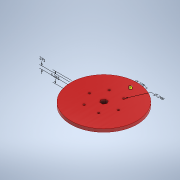
# Autodesk Inventor part: attachementToTripod
Saved by Autodesk Inventor 2022.2 (Build 262287010, 287A)
## iProperties
Created: 2021-02-15
Part Number: attachementToTripod
Material: PC/ABS Plastic
Document SubType Name: Modeling
Designer: robst
Density: 0.357273 g/cm^3
Appearance: Red
Author: robst
Autodesk Inventor part; units mm, degrees
(part 1 of 2)
ref_plane "YZ Plane" through (0, 0, 0) normal (1, 0, 0) x (0, 1, 0)
ref_plane "XZ Plane" through (0, 0, 0) normal (0, 1, 0) x (-1, 0, 0)
ref_plane "XY Plane" through (0, 0, 0) normal (0, 0, 1) x (1, 0, 0)
sketch "Sketch2" plane through (0, 0, 0) normal (0, 0, 1) x (1, 0, 0)
  line L0 (-101.6, 0) -> (-101.6, -9.525)
  line L1 (-101.6, -9.525) -> (-12.7, -9.525)
  line L2 (-10.795, -44.525) -> (0, -44.525)
  line L3 (-101.6, 0) -> (0, 0)
  line L4 (0, 0) -> (0, -44.525) construction
  line L5 (0, 0) -> (0, -44.525)
  line L6 (0, -53.43) -> (0, 8.905) projected
  line L7 (-12.7, -9.525) -> (-10.795, -44.525)
  dimension "d0" = 101.6
  dimension "d3" = 9.525
  dimension "d4" = 35
  dimension "d64" = 10.795
  constraints: 14 end point, 3 vertical, 2 horizontal, 1 perpendicular
  measures "d0" distance from line of L0 L3.end
  measures "d3" distance from line of L1 L3.end
  measures "d4" distance from line of L2.start L1
  measures "d64" horizontal distance of L2.start L3.end
revolve "Revolution1" add sketch "Sketch2" angle 360 about axis through (0, -10, 0) along (0, 1, 0)
sketch "Sketch5" plane through (0, -9.525, 0) normal (0, -1, 0) x (1, 0, 0)
  circle A0 centre (0, 0) radius 76.2 construction
  line L0 (6.8814, -79.1482) -> (6.9305, -79.1427)
  spline S0 degree 2 poles (6.9305, -79.1427) (7.0648, -79.1774) (7.5531, -79.21) (7.7433, -79.1888) knots 0 0 0 1 2 2 2
  spline S1 degree 2 poles (7.7433, -79.1888) (8.3448, -79.1218) (8.8001, -78.5243) (8.7208, -77.8124) knots 0 0 0 1 2 2 2
  line L1 (8.7208, -77.8124) -> (8.6996, -77.6221)
  line L2 (8.6996, -77.6221) -> (7.1162, -77.7986)
  line L3 (7.1162, -77.7986) -> (7.028, -77.0069)
  line L4 (7.028, -77.0069) -> (8.5807, -76.8339)
  line L5 (8.5807, -76.8339) -> (8.0356, -71.9426)
  line L6 (8.0356, -71.9426) -> (8.993, -71.8359)
  line L7 (8.993, -71.8359) -> (9.5381, -76.7272)
  line L8 (9.5381, -76.7272) -> (10.1824, -76.6554)
  line L9 (10.1824, -76.6554) -> (10.2707, -77.447)
  line L10 (10.2707, -77.447) -> (9.6263, -77.5189)
  line L11 (9.6263, -77.5189) -> (9.6475, -77.7091)
  spline S2 degree 2 poles (9.6475, -77.7091) (9.761, -78.7279) (8.8919, -79.9058) (7.9714, -80.0084) knots 0 0 0 1 2 2 2
  spline S3 degree 2 poles (7.9714, -80.0084) (7.7075, -80.0378) (7.1919, -80.0393) (6.9792, -80.0258) knots 0 0 0 1 2 2 2
  line L12 (6.9792, -80.0258) -> (6.8814, -79.1482)
  line L13 (4.5732, -72.247) -> (5.5341, -72.1798)
  line L14 (5.5341, -72.1798) -> (5.9333, -77.8839)
  line L15 (5.9333, -77.8839) -> (4.9724, -77.9511)
  line L16 (4.9724, -77.9511) -> (4.5732, -72.247)
  line L17 (4.971, -78.9045) -> (6.0613, -78.8282)
  line L18 (6.0613, -78.8282) -> (6.1312, -79.8261)
  line L19 (6.1312, -79.8261) -> (5.0408, -79.9024)
  line L20 (5.0408, -79.9024) -> (4.971, -78.9045)
  line L21 (2.1802, -72.3588) -> (3.1428, -72.3233)
  line L22 (3.1428, -72.3233) -> (3.4355, -80.2776)
  line L23 (3.4355, -80.2776) -> (2.4728, -80.313)
  line L24 (2.4728, -80.313) -> (2.1802, -72.3588)
  spline S4 degree 2 poles (-1.7121, -72.2413) (-0.3415, -72.2657) (1.1375, -73.83) (1.1122, -75.25) knots 0 0 0 1 2 2 2
  spline S5 degree 2 poles (1.1122, -75.25) (1.0873, -76.6453) (-0.4055, -78.2739) (-1.5847, -78.2528) knots 0 0 0 1 2 2 2
  spline S6 degree 2 poles (-1.5847, -78.2528) (-2.1157, -78.2433) (-2.9313, -77.92) (-3.228, -77.5874) knots 0 0 0 1 2 2 2
  spline S7 degree 2 poles (-3.228, -77.5874) (-3.5309, -77.2546) (-3.8412, -76.3042) (-3.829, -75.6188) knots 0 0 0 1 2 2 2
  line L25 (-3.829, -75.6188) -> (-3.8196, -75.094)
  line L26 (-3.8196, -75.094) -> (0.1379, -75.1647)
  spline S8 degree 2 poles (0.1379, -75.1647) (0.1557, -74.1706) (-0.8257, -73.097) (-1.7148, -73.0812) knots 0 0 0 1 2 2 2
  spline S9 degree 2 poles (-1.7148, -73.0812) (-2.0296, -73.0755) (-2.6434, -73.2066) (-2.8924, -73.3134) knots 0 0 0 1 2 2 2
  spline S10 degree 2 poles (-2.8924, -73.3134) (-3.1539, -73.4322) (-3.5158, -73.6419) (-3.6349, -73.7386) knots 0 0 0 1 2 2 2
  line L27 (-3.6349, -73.7386) -> (-3.6905, -73.7376)
  line L28 (-3.6905, -73.7376) -> (-3.6717, -72.688)
  spline S11 degree 2 poles (-3.6717, -72.688) (-3.5038, -72.6231) (-2.994, -72.4346) (-2.7955, -72.3825) knots 0 0 0 1 2 2 2
  spline S12 degree 2 poles (-2.7955, -72.3825) (-2.5162, -72.3072) (-2.0579, -72.2351) (-1.7121, -72.2413) knots 0 0 0 1 2 2 2
  spline S13 degree 2 poles (-2.8943, -75.8455) (-2.8889, -76.2347) (-2.7385, -76.8056) (-2.5876, -76.9997) knots 0 0 0 1 2 2 2
  spline S14 degree 2 poles (-2.5876, -76.9997) (-2.4247, -77.2188) (-1.904, -77.4566) (-1.515, -77.4635) knots 0 0 0 1 2 2 2
  spline S15 degree 2 poles (-1.515, -77.4635) (-1.1323, -77.4704) (-0.591, -77.2515) (-0.3648, -77.0332) knots 0 0 0 1 2 2 2
  spline S16 degree 2 poles (-0.3648, -77.0332) (-0.1446, -76.8086) (0.0874, -76.2631) (0.1248, -75.8994) knots 0 0 0 1 2 2 2
  line L29 (0.1248, -75.8994) -> (-2.8943, -75.8455)
  line L30 (-6.5023, -72.1) -> (-5.2837, -72.1995)
  line L31 (-5.2837, -72.1995) -> (-5.4023, -73.652)
  line L32 (-5.4023, -73.652) -> (-6.6209, -73.5524)
  line L33 (-6.6209, -73.5524) -> (-6.5023, -72.1)
  line L34 (-6.8491, -76.3466) -> (-5.6305, -76.4461)
  line L35 (-5.6305, -76.4461) -> (-5.7492, -77.8986)
  line L36 (-5.7492, -77.8986) -> (-6.9678, -77.7991)
  line L37 (-6.9678, -77.7991) -> (-6.8491, -76.3466)
  spline S17 degree 2 poles (-14.9177, -71.4636) (-14.7861, -71.4009) (-14.3396, -71.1724) (-14.1402, -71.1165) knots 0 0 0 1 2 2 2
  spline S18 degree 2 poles (-14.1402, -71.1165) (-13.8659, -71.031) (-13.3722, -70.9814) (-12.9477, -71.0632) knots 0 0 0 1 2 2 2
  spline S19 degree 2 poles (-12.9477, -71.0632) (-12.6021, -71.1298) (-12.0277, -71.5108) (-11.8368, -71.7928) knots 0 0 0 1 2 2 2
  spline S20 degree 2 poles (-11.8368, -71.7928) (-11.6568, -72.0664) (-11.5148, -72.7981) (-11.5872, -73.174) knots 0 0 0 1 2 2 2
  spline S21 degree 2 poles (-11.5872, -73.174) (-11.6993, -73.7562) (-12.3493, -74.4862) (-12.9284, -74.6199) knots 0 0 0 1 2 2 2
  spline S22 degree 2 poles (-12.9284, -74.6199) (-13.4434, -74.7471) (-14.7604, -74.6633) (-15.5144, -74.5621) knots 0 0 0 1 2 2 2
  line L38 (-15.5144, -74.5621) -> (-15.5495, -74.744)
  spline S23 degree 2 poles (-15.5495, -74.744) (-15.6125, -75.0714) (-15.4907, -75.5162) (-15.331, -75.6664) knots 0 0 0 1 2 2 2
  spline S24 degree 2 poles (-15.331, -75.6664) (-15.1712, -75.8167) (-14.6638, -75.9899) (-14.3849, -76.0436) knots 0 0 0 1 2 2 2
  spline S25 degree 2 poles (-14.3849, -76.0436) (-14.0574, -76.1067) (-13.1348, -76.0831) (-12.6559, -75.9804) knots 0 0 0 1 2 2 2
  line L39 (-12.6559, -75.9804) -> (-12.6013, -75.9909)
  line L40 (-12.6013, -75.9909) -> (-12.787, -76.955)
  spline S26 degree 2 poles (-12.787, -76.955) (-13.0618, -76.9776) (-14.0731, -76.9715) (-14.5521, -76.8792) knots 0 0 0 1 2 2 2
  spline S27 degree 2 poles (-14.5521, -76.8792) (-15.1342, -76.7671) (-15.8935, -76.4322) (-16.1632, -76.135) knots 0 0 0 1 2 2 2
  spline S28 degree 2 poles (-16.1632, -76.135) (-16.4281, -75.845) (-16.59, -75.0529) (-16.4884, -74.5254) knots 0 0 0 1 2 2 2
  line L41 (-16.4884, -74.5254) -> (-15.7491, -70.6871)
  line L42 (-15.7491, -70.6871) -> (-14.8032, -70.8693)
  line L43 (-14.8032, -70.8693) -> (-14.9177, -71.4636)
  line L44 (-15.0695, -72.2518) -> (-15.3696, -73.8102)
  spline S29 degree 2 poles (-15.3696, -73.8102) (-15.0242, -73.8453) (-13.9796, -73.9395) (-13.6396, -73.9044) knots 0 0 0 1 2 2 2
  spline S30 degree 2 poles (-13.6396, -73.9044) (-13.2414, -73.8616) (-12.658, -73.4772) (-12.5763, -73.0527) knots 0 0 0 1 2 2 2
  spline S31 degree 2 poles (-12.5763, -73.0527) (-12.4828, -72.5676) (-12.934, -71.9714) (-13.4554, -71.8709) knots 0 0 0 1 2 2 2
  spline S32 degree 2 poles (-13.4554, -71.8709) (-13.8981, -71.7857) (-14.6993, -72.0276) (-15.0695, -72.2518) knots 0 0 0 1 2 2 2
  spline S33 degree 2 poles (-18.707, -69.8193) (-17.9476, -70.0152) (-17.3162, -71.1028) (-17.5584, -72.0415) knots 0 0 0 1 2 2 2
  line L45 (-17.5584, -72.0415) -> (-18.3497, -75.1089)
  line L46 (-18.3497, -75.1089) -> (-17.7219, -75.2709)
  line L47 (-17.7219, -75.2709) -> (-17.9209, -76.0422)
  line L48 (-17.9209, -76.0422) -> (-18.5487, -75.8802)
  line L49 (-18.5487, -75.8802) -> (-18.959, -77.4707)
  line L50 (-18.959, -77.4707) -> (-19.8918, -77.2301)
  line L51 (-19.8918, -77.2301) -> (-19.4815, -75.6396)
  line L52 (-19.4815, -75.6396) -> (-21.1975, -75.1969)
  line L53 (-21.1975, -75.1969) -> (-20.9985, -74.4256)
  line L54 (-20.9985, -74.4256) -> (-19.2825, -74.8683)
  line L55 (-19.2825, -74.8683) -> (-18.6022, -72.2314)
  spline S34 degree 2 poles (-18.6022, -72.2314) (-18.4942, -71.8129) (-18.4054, -71.3447) (-18.4561, -71.1212) knots 0 0 0 1 2 2 2
  spline S35 degree 2 poles (-18.4561, -71.1212) (-18.4951, -70.9262) (-18.827, -70.6556) (-19.1499, -70.5723) knots 0 0 0 1 2 2 2
  spline S36 degree 2 poles (-19.1499, -70.5723) (-19.3771, -70.5137) (-19.8371, -70.5417) (-19.9436, -70.5589) knots 0 0 0 1 2 2 2
  line L56 (-19.9436, -70.5589) -> (-19.9974, -70.545)
  line L57 (-19.9974, -70.545) -> (-19.7815, -69.7079)
  spline S37 degree 2 poles (-19.7815, -69.7079) (-19.4999, -69.704) (-18.9401, -69.7591) (-18.707, -69.8193) knots 0 0 0 1 2 2 2
  spline S38 degree 2 poles (-22.0659, -68.8315) (-21.3169, -69.064) (-20.7389, -70.1809) (-21.0263, -71.1068) knots 0 0 0 1 2 2 2
  line L58 (-21.0263, -71.1068) -> (-21.9652, -74.1322)
  line L59 (-21.9652, -74.1322) -> (-21.346, -74.3244)
  line L60 (-21.346, -74.3244) -> (-21.5821, -75.0852)
  line L61 (-21.5821, -75.0852) -> (-22.2013, -74.893)
  line L62 (-22.2013, -74.893) -> (-22.6881, -76.4618)
  line L63 (-22.6881, -76.4618) -> (-23.6082, -76.1763)
  line L64 (-23.6082, -76.1763) -> (-23.1213, -74.6075)
  line L65 (-23.1213, -74.6075) -> (-24.8139, -74.0822)
  line L66 (-24.8139, -74.0822) -> (-24.5778, -73.3214)
  line L67 (-24.5778, -73.3214) -> (-22.8852, -73.8467)
  line L68 (-22.8852, -73.8467) -> (-22.0781, -71.2459)
  spline S39 degree 2 poles (-22.0781, -71.2459) (-21.95, -70.8331) (-21.8385, -70.3698) (-21.8784, -70.1441) knots 0 0 0 1 2 2 2
  spline S40 degree 2 poles (-21.8784, -70.1441) (-21.9079, -69.9474) (-22.2263, -69.6611) (-22.5448, -69.5622) knots 0 0 0 1 2 2 2
  spline S41 degree 2 poles (-22.5448, -69.5622) (-22.7689, -69.4927) (-23.2297, -69.4984) (-23.3369, -69.5104) knots 0 0 0 1 2 2 2
  line L69 (-23.3369, -69.5104) -> (-23.39, -69.4939)
  line L70 (-23.39, -69.4939) -> (-23.1338, -68.6682)
  spline S42 degree 2 poles (-23.1338, -68.6682) (-22.8523, -68.678) (-22.2959, -68.7602) (-22.0659, -68.8315) knots 0 0 0 1 2 2 2
  spline S43 degree 2 poles (-26.9866, -67.8329) (-26.8462, -67.7937) (-26.3671, -67.6455) (-26.161, -67.6247) knots 0 0 0 1 2 2 2
  spline S44 degree 2 poles (-26.161, -67.6247) (-25.8761, -67.5876) (-25.3812, -67.6238) (-24.9771, -67.7773) knots 0 0 0 1 2 2 2
  spline S45 degree 2 poles (-24.9771, -67.7773) (-24.6481, -67.9023) (-24.1479, -68.3764) (-24.0083, -68.6871) knots 0 0 0 1 2 2 2
  spline S46 degree 2 poles (-24.0083, -68.6871) (-23.8781, -68.9876) (-23.8639, -69.7328) (-23.9999, -70.0907) knots 0 0 0 1 2 2 2
  spline S47 degree 2 poles (-23.9999, -70.0907) (-24.2105, -70.6449) (-24.9763, -71.2522) (-25.5699, -71.2844) knots 0 0 0 1 2 2 2
  spline S48 degree 2 poles (-25.5699, -71.2844) (-26.0991, -71.3211) (-27.382, -71.0119) (-28.1074, -70.7826) knots 0 0 0 1 2 2 2
  line L71 (-28.1074, -70.7826) -> (-28.1732, -70.9557)
  spline S49 degree 2 poles (-28.1732, -70.9557) (-28.2916, -71.2675) (-28.2481, -71.7266) (-28.1166, -71.9021) knots 0 0 0 1 2 2 2
  spline S50 degree 2 poles (-28.1166, -71.9021) (-27.9851, -72.0775) (-27.515, -72.3354) (-27.2495, -72.4363) knots 0 0 0 1 2 2 2
  spline S51 degree 2 poles (-27.2495, -72.4363) (-26.9378, -72.5548) (-26.0248, -72.6903) (-25.5354, -72.6714) knots 0 0 0 1 2 2 2
  line L72 (-25.5354, -72.6714) -> (-25.4835, -72.6912)
  line L73 (-25.4835, -72.6912) -> (-25.8322, -73.609)
  spline S52 degree 2 poles (-25.8322, -73.609) (-26.1067, -73.5839) (-27.1019, -73.404) (-27.5579, -73.2307) knots 0 0 0 1 2 2 2
  spline S53 degree 2 poles (-27.5579, -73.2307) (-28.1121, -73.0202) (-28.8024, -72.5597) (-29.0171, -72.2205) knots 0 0 0 1 2 2 2
  spline S54 degree 2 poles (-29.0171, -72.2205) (-29.2281, -71.8893) (-29.2513, -71.0811) (-29.0605, -70.579) knots 0 0 0 1 2 2 2
  line L74 (-29.0605, -70.579) -> (-27.6721, -66.925)
  line L75 (-27.6721, -66.925) -> (-26.7716, -67.2672)
  line L76 (-26.7716, -67.2672) -> (-26.9866, -67.8329)
  line L77 (-27.2717, -68.5833) -> (-27.8354, -70.0668)
  spline S55 degree 2 poles (-27.8354, -70.0668) (-27.5012, -70.1608) (-26.4884, -70.4333) (-26.1473, -70.4572) knots 0 0 0 1 2 2 2
  spline S56 degree 2 poles (-26.1473, -70.4572) (-25.7478, -70.4835) (-25.1069, -70.2051) (-24.9534, -69.8011) knots 0 0 0 1 2 2 2
  spline S57 degree 2 poles (-24.9534, -69.8011) (-24.7779, -69.3393) (-25.1198, -68.6743) (-25.6162, -68.4857) knots 0 0 0 1 2 2 2
  spline S58 degree 2 poles (-25.6162, -68.4857) (-26.0376, -68.3256) (-26.8685, -68.426) (-27.2717, -68.5833) knots 0 0 0 1 2 2 2
  spline S59 degree 2 poles (-30.919, -65.3137) (-30.3813, -65.5632) (-29.644, -66.307) (-29.4807, -66.7912) knots 0 0 0 1 2 2 2
  spline S60 degree 2 poles (-29.4807, -66.7912) (-29.3148, -67.2699) (-29.435, -68.4531) (-29.7521, -69.1364) knots 0 0 0 1 2 2 2
  spline S61 degree 2 poles (-29.7521, -69.1364) (-30.0693, -69.8198) (-30.896, -70.6478) (-31.3601, -70.841) knots 0 0 0 1 2 2 2
  spline S62 degree 2 poles (-31.3601, -70.841) (-31.8267, -71.0397) (-32.9087, -70.9801) (-33.4352, -70.7357) knots 0 0 0 1 2 2 2
  spline S63 degree 2 poles (-33.4352, -70.7357) (-33.8609, -70.5382) (-34.5445, -69.9282) (-34.7798, -69.6284) knots 0 0 0 1 2 2 2
  line L78 (-34.7798, -69.6284) -> (-34.3249, -68.6482)
  line L79 (-34.3249, -68.6482) -> (-34.2745, -68.6716)
  spline S64 degree 2 poles (-34.2745, -68.6716) (-34.2156, -68.7942) (-34.018, -69.131) (-33.8601, -69.3336) knots 0 0 0 1 2 2 2
  spline S65 degree 2 poles (-33.8601, -69.3336) (-33.7168, -69.509) (-33.2889, -69.8778) (-33.0649, -69.9817) knots 0 0 0 1 2 2 2
  spline S66 degree 2 poles (-33.0649, -69.9817) (-32.3871, -70.2963) (-31.088, -69.6533) (-30.6539, -68.7179) knots 0 0 0 1 2 2 2
  spline S67 degree 2 poles (-30.6539, -68.7179) (-30.2302, -67.8049) (-30.5499, -66.4108) (-31.2557, -66.0832) knots 0 0 0 1 2 2 2
  spline S68 degree 2 poles (-31.2557, -66.0832) (-31.6814, -65.8857) (-32.6181, -65.8799) (-33.0424, -66.0166) knots 0 0 0 1 2 2 2
  line L80 (-33.0424, -66.0166) -> (-33.0928, -65.9932)
  line L81 (-33.0928, -65.9932) -> (-32.6379, -65.0129)
  spline S69 degree 2 poles (-32.6379, -65.0129) (-32.4805, -65.0111) (-32.0078, -65.0194) (-31.8328, -65.053) knots 0 0 0 1 2 2 2
  spline S70 degree 2 poles (-31.8328, -65.053) (-31.5775, -65.0898) (-31.1935, -65.1863) (-30.919, -65.3137) knots 0 0 0 1 2 2 2
  line L82 (-37.2051, -62.1388) -> (-36.3635, -62.6076)
  line L83 (-36.3635, -62.6076) -> (-37.95, -65.4559)
  spline S71 degree 2 poles (-37.95, -65.4559) (-38.1423, -65.8012) (-38.4081, -66.4307) (-38.4102, -66.6628) knots 0 0 0 1 2 2 2
  spline S72 degree 2 poles (-38.4102, -66.6628) (-38.4128, -66.9087) (-38.1482, -67.2964) (-37.8353, -67.4707) knots 0 0 0 1 2 2 2
  spline S73 degree 2 poles (-37.8353, -67.4707) (-37.5224, -67.645) (-36.6725, -67.6801) (-36.204, -67.5877) knots 0 0 0 1 2 2 2
  line L84 (-36.204, -67.5877) -> (-34.1247, -63.8545)
  line L85 (-34.1247, -63.8545) -> (-33.2831, -64.3233)
  line L86 (-33.2831, -64.3233) -> (-37.1563, -71.277)
  line L87 (-37.1563, -71.277) -> (-37.9979, -70.8083)
  line L88 (-37.9979, -70.8083) -> (-36.5977, -68.2944)
  spline S74 degree 2 poles (-36.5977, -68.2944) (-37.1646, -68.4239) (-38.0912, -68.3743) (-38.5012, -68.1459) knots 0 0 0 1 2 2 2
  spline S75 degree 2 poles (-38.5012, -68.1459) (-39.2348, -67.7373) (-39.5248, -66.3035) (-39.0109, -65.381) knots 0 0 0 1 2 2 2
  line L89 (-39.0109, -65.381) -> (-37.2051, -62.1388)
  spline S76 degree 2 poles (-40.3503, -59.9465) (-39.2086, -60.7053) (-38.8049, -62.8199) (-39.591, -64.0027) knots 0 0 0 1 2 2 2
  spline S77 degree 2 poles (-39.591, -64.0027) (-40.3635, -65.165) (-42.4984, -65.7332) (-43.4806, -65.0803) knots 0 0 0 1 2 2 2
  spline S78 degree 2 poles (-43.4806, -65.0803) (-43.9229, -64.7864) (-44.436, -64.0746) (-44.5068, -63.6346) knots 0 0 0 1 2 2 2
  spline S79 degree 2 poles (-44.5068, -63.6346) (-44.5828, -63.1911) (-44.3324, -62.2231) (-43.953, -61.6523) knots 0 0 0 1 2 2 2
  line L90 (-43.953, -61.6523) -> (-43.6625, -61.2151)
  line L91 (-43.6625, -61.2151) -> (-40.366, -63.4061)
  spline S80 degree 2 poles (-40.366, -63.4061) (-39.8157, -62.5781) (-40.0643, -61.145) (-40.8049, -60.6528) knots 0 0 0 1 2 2 2
  spline S81 degree 2 poles (-40.8049, -60.6528) (-41.0671, -60.4785) (-41.6549, -60.2584) (-41.9221, -60.2142) knots 0 0 0 1 2 2 2
  spline S82 degree 2 poles (-41.9221, -60.2142) (-42.2065, -60.1735) (-42.6244, -60.1553) (-42.7768, -60.1726) knots 0 0 0 1 2 2 2
  line L92 (-42.7768, -60.1726) -> (-42.8231, -60.1418)
  line L93 (-42.8231, -60.1418) -> (-42.242, -59.2676)
  spline S83 degree 2 poles (-42.242, -59.2676) (-42.0656, -59.3033) (-41.5345, -59.419) (-41.3391, -59.4821) knots 0 0 0 1 2 2 2
  spline S84 degree 2 poles (-41.3391, -59.4821) (-41.0633, -59.569) (-40.6383, -59.7551) (-40.3503, -59.9465) knots 0 0 0 1 2 2 2
  spline S85 degree 2 poles (-43.2875, -62.3467) (-43.4926, -62.6775) (-43.6733, -63.2395) (-43.6507, -63.4844) knots 0 0 0 1 2 2 2
  spline S86 degree 2 poles (-43.6507, -63.4844) (-43.6315, -63.7567) (-43.3208, -64.2375) (-42.9968, -64.4528) knots 0 0 0 1 2 2 2
  spline S87 degree 2 poles (-42.9968, -64.4528) (-42.678, -64.6647) (-42.1041, -64.7718) (-41.7959, -64.7097) knots 0 0 0 1 2 2 2
  spline S88 degree 2 poles (-41.7959, -64.7097) (-41.4894, -64.6391) (-41.0001, -64.3044) (-40.7727, -64.0181) knots 0 0 0 1 2 2 2
  line L94 (-40.7727, -64.0181) -> (-43.2875, -62.3467)
  line L95 (-47.9733, -54.2827) -> (-50.0683, -56.8451)
  spline S89 degree 2 poles (-50.0683, -56.8451) (-50.3185, -57.1511) (-50.6967, -57.7112) (-50.7375, -57.9172) knots 0 0 0 1 2 2 2
  spline S90 degree 2 poles (-50.7375, -57.9172) (-50.7899, -58.1375) (-50.6234, -58.5289) (-50.37, -58.736) knots 0 0 0 1 2 2 2
  spline S91 degree 2 poles (-50.37, -58.736) (-50.1406, -58.9236) (-49.3841, -59.0715) (-48.8879, -59.0305) knots 0 0 0 1 2 2 2
  spline S92 degree 2 poles (-48.8879, -59.0305) (-48.838, -58.9597) (-48.6951, -58.7654) (-48.5935, -58.6411) knots 0 0 0 1 2 2 2
  line L96 (-48.5935, -58.6411) -> (-46.2093, -55.7249)
  line L97 (-46.2093, -55.7249) -> (-45.4635, -56.3347)
  line L98 (-45.4635, -56.3347) -> (-47.5585, -58.8971)
  spline S93 degree 2 poles (-47.5585, -58.8971) (-47.8086, -59.203) (-48.1869, -59.7632) (-48.2276, -59.9692) knots 0 0 0 1 2 2 2
  spline S94 degree 2 poles (-48.2276, -59.9692) (-48.2801, -60.1895) (-48.1136, -60.5809) (-47.8602, -60.788) knots 0 0 0 1 2 2 2
  spline S95 degree 2 poles (-47.8602, -60.788) (-47.6212, -60.9834) (-46.8443, -61.1161) (-46.4042, -61.0851) knots 0 0 0 1 2 2 2
  line L99 (-46.4042, -61.0851) -> (-43.6995, -57.7769)
  line L100 (-43.6995, -57.7769) -> (-42.9537, -58.3866)
  line L101 (-42.9537, -58.3866) -> (-46.573, -62.8135)
  line L102 (-46.573, -62.8135) -> (-47.3188, -62.2038)
  line L103 (-47.3188, -62.2038) -> (-46.9201, -61.7161)
  spline S96 degree 2 poles (-46.9201, -61.7161) (-47.4501, -61.7693) (-48.2857, -61.6206) (-48.6299, -61.3392) knots 0 0 0 1 2 2 2
  spline S97 degree 2 poles (-48.6299, -61.3392) (-49.0219, -61.0187) (-49.3359, -60.1638) (-49.1614, -59.6284) knots 0 0 0 1 2 2 2
  spline S98 degree 2 poles (-49.1614, -59.6284) (-49.8096, -59.7286) (-50.7668, -59.5921) (-51.1397, -59.2872) knots 0 0 0 1 2 2 2
  spline S99 degree 2 poles (-51.1397, -59.2872) (-51.4266, -59.0527) (-51.7504, -58.4928) (-51.7584, -58.1513) knots 0 0 0 1 2 2 2
  spline S100 degree 2 poles (-51.7584, -58.1513) (-51.7711, -57.8059) (-51.4746, -57.0433) (-51.1033, -56.5891) knots 0 0 0 1 2 2 2
  line L104 (-51.1033, -56.5891) -> (-48.7191, -53.6729)
  line L105 (-48.7191, -53.6729) -> (-47.9733, -54.2827)
  spline S101 degree 2 poles (-51.3308, -50.8614) (-50.3602, -51.8295) (-50.3793, -53.9822) (-51.3824, -54.9877) knots 0 0 0 1 2 2 2
  spline S102 degree 2 poles (-51.3824, -54.9877) (-52.3679, -55.9758) (-54.5728, -56.1139) (-55.4078, -55.281) knots 0 0 0 1 2 2 2
  spline S103 degree 2 poles (-55.4078, -55.281) (-55.7838, -54.906) (-56.1472, -54.1074) (-56.1303, -53.662) knots 0 0 0 1 2 2 2
  spline S104 degree 2 poles (-56.1303, -53.662) (-56.1178, -53.2122) (-55.6823, -52.3122) (-55.1982, -51.8269) knots 0 0 0 1 2 2 2
  line L106 (-55.1982, -51.8269) -> (-54.8275, -51.4553)
  line L107 (-54.8275, -51.4553) -> (-52.0251, -54.2506)
  spline S105 degree 2 poles (-52.0251, -54.2506) (-51.323, -53.5467) (-51.2856, -52.0927) (-51.9151, -51.4647) knots 0 0 0 1 2 2 2
  spline S106 degree 2 poles (-51.9151, -51.4647) (-52.1381, -51.2423) (-52.6712, -50.9111) (-52.9246, -50.8154) knots 0 0 0 1 2 2 2
  spline S107 degree 2 poles (-52.9246, -50.8154) (-53.1954, -50.7197) (-53.6016, -50.6198) (-53.7545, -50.6068) knots 0 0 0 1 2 2 2
  line L108 (-53.7545, -50.6068) -> (-53.7938, -50.5676)
  line L109 (-53.7938, -50.5676) -> (-53.0525, -49.8244)
  spline S108 degree 2 poles (-53.0525, -49.8244) (-52.8865, -49.894) (-52.3884, -50.1117) (-52.2093, -50.2119) knots 0 0 0 1 2 2 2
  spline S109 degree 2 poles (-52.2093, -50.2119) (-51.9558, -50.3513) (-51.5756, -50.6172) (-51.3308, -50.8614) knots 0 0 0 1 2 2 2
  spline S110 degree 2 poles (-54.682, -52.6384) (-54.948, -52.9226) (-55.2355, -53.4382) (-55.2614, -53.6827) knots 0 0 0 1 2 2 2
  spline S111 degree 2 poles (-55.2614, -53.6827) (-55.296, -53.9535) (-55.0857, -54.4859) (-54.8103, -54.7606) knots 0 0 0 1 2 2 2
  spline S112 degree 2 poles (-54.8103, -54.7606) (-54.5392, -55.031) (-53.9975, -55.2487) (-53.6831, -55.2483) knots 0 0 0 1 2 2 2
  spline S113 degree 2 poles (-53.6831, -55.2483) (-53.3688, -55.2391) (-52.8232, -55.007) (-52.5441, -54.7709) knots 0 0 0 1 2 2 2
  line L110 (-52.5441, -54.7709) -> (-54.682, -52.6384)
  line L111 (-56.4539, -45.3697) -> (-55.8273, -46.1013)
  line L112 (-55.8273, -46.1013) -> (-58.3035, -48.2222)
  spline S114 degree 2 poles (-58.3035, -48.2222) (-58.6037, -48.4793) (-59.0714, -48.9775) (-59.1538, -49.1944) knots 0 0 0 1 2 2 2
  spline S115 degree 2 poles (-59.1538, -49.1944) (-59.2416, -49.4241) (-59.1279, -49.8796) (-58.895, -50.1516) knots 0 0 0 1 2 2 2
  spline S116 degree 2 poles (-58.895, -50.1516) (-58.662, -50.4237) (-57.8771, -50.7515) (-57.4056, -50.8273) knots 0 0 0 1 2 2 2
  line L113 (-57.4056, -50.8273) -> (-54.1602, -48.0476)
  line L114 (-54.1602, -48.0476) -> (-53.5336, -48.7792)
  line L115 (-53.5336, -48.7792) -> (-57.8764, -52.4989)
  line L116 (-57.8764, -52.4989) -> (-58.5031, -51.7673)
  line L117 (-58.5031, -51.7673) -> (-58.02, -51.3535)
  spline S117 degree 2 poles (-58.02, -51.3535) (-58.5967, -51.2783) (-59.4485, -50.9103) (-59.7538, -50.5539) knots 0 0 0 1 2 2 2
  spline S118 degree 2 poles (-59.7538, -50.5539) (-60.3001, -49.916) (-60.0745, -48.4707) (-59.2725, -47.7838) knots 0 0 0 1 2 2 2
  line L118 (-59.2725, -47.7838) -> (-56.4539, -45.3697)
  spline S119 degree 2 poles (-58.2177, -42.8414) (-57.747, -43.4686) (-57.9333, -44.7123) (-58.7087, -45.2942) knots 0 0 0 1 2 2 2
  line L119 (-58.7087, -45.2942) -> (-61.2425, -47.1954)
  line L120 (-61.2425, -47.1954) -> (-60.8534, -47.714)
  line L121 (-60.8534, -47.714) -> (-61.4906, -48.1921)
  line L122 (-61.4906, -48.1921) -> (-61.8797, -47.6735)
  line L123 (-61.8797, -47.6735) -> (-63.1935, -48.6593)
  line L124 (-63.1935, -48.6593) -> (-63.7717, -47.8888)
  line L125 (-63.7717, -47.8888) -> (-62.4579, -46.903)
  line L126 (-62.4579, -46.903) -> (-63.5215, -45.4854)
  line L127 (-63.5215, -45.4854) -> (-62.8843, -45.0073)
  line L128 (-62.8843, -45.0073) -> (-61.8207, -46.4249)
  line L129 (-61.8207, -46.4249) -> (-59.6425, -44.7905)
  spline S120 degree 2 poles (-59.6425, -44.7905) (-59.2967, -44.5311) (-58.935, -44.221) (-58.835, -44.0148) knots 0 0 0 1 2 2 2
  spline S121 degree 2 poles (-58.835, -44.0148) (-58.7436, -43.8381) (-58.8339, -43.4195) (-59.034, -43.1528) knots 0 0 0 1 2 2 2
  spline S122 degree 2 poles (-59.034, -43.1528) (-59.1748, -42.9651) (-59.5516, -42.6996) (-59.6454, -42.6465) knots 0 0 0 1 2 2 2
  line L130 (-59.6454, -42.6465) -> (-59.6788, -42.6021)
  line L131 (-59.6788, -42.6021) -> (-58.9873, -42.0832)
  spline S123 degree 2 poles (-58.9873, -42.0832) (-58.765, -42.2561) (-58.3623, -42.6487) (-58.2177, -42.8414) knots 0 0 0 1 2 2 2
  line L132 (-60.3823, -39.9319) -> (-66.0123, -43.598)
  line L133 (-66.0123, -43.598) -> (-64.6172, -45.7403)
  line L134 (-64.6172, -45.7403) -> (-65.3727, -46.2323)
  line L135 (-65.3727, -46.2323) -> (-68.7154, -41.0991)
  line L136 (-68.7154, -41.0991) -> (-67.9599, -40.6071)
  line L137 (-67.9599, -40.6071) -> (-66.5649, -42.7494)
  line L138 (-66.5649, -42.7494) -> (-60.9349, -39.0832)
  line L139 (-60.9349, -39.0832) -> (-60.3823, -39.9319)
  spline S124 degree 2 poles (-67.4075, -33.5435) (-66.1364, -32.8563) (-64.0905, -33.3296) (-63.5383, -34.3507) knots 0 0 0 1 2 2 2
  spline S125 degree 2 poles (-63.5383, -34.3507) (-62.9715, -35.3991) (-63.751, -37.372) (-64.9786, -38.0357) knots 0 0 0 1 2 2 2
  spline S126 degree 2 poles (-64.9786, -38.0357) (-66.2388, -38.7171) (-68.3045, -38.2334) (-68.8507, -37.2231) knots 0 0 0 1 2 2 2
  spline S127 degree 2 poles (-68.8507, -37.2231) (-69.4029, -36.2019) (-68.6731, -34.2279) (-67.4075, -33.5435) knots 0 0 0 1 2 2 2
  spline S128 degree 2 poles (-66.9346, -34.4181) (-67.9124, -34.9467) (-68.4782, -36.1723) (-68.1228, -36.8295) knots 0 0 0 1 2 2 2
  spline S129 degree 2 poles (-68.1228, -36.8295) (-67.7675, -37.4868) (-66.4292, -37.6898) (-65.4515, -37.1612) knots 0 0 0 1 2 2 2
  spline S130 degree 2 poles (-65.4515, -37.1612) (-64.5009, -36.6472) (-63.9108, -35.4016) (-64.2662, -34.7443) knots 0 0 0 1 2 2 2
  spline S131 degree 2 poles (-64.2662, -34.7443) (-64.6186, -34.0925) (-65.9678, -33.8953) (-66.9346, -34.4181) knots 0 0 0 1 2 2 2
  line L140 (-66.0648, -29.5977) -> (-72.2153, -32.301)
  line L141 (-72.2153, -32.301) -> (-71.1866, -34.6414)
  line L142 (-71.1866, -34.6414) -> (-72.012, -35.0042)
  line L143 (-72.012, -35.0042) -> (-74.4768, -29.3963)
  line L144 (-74.4768, -29.3963) -> (-73.6515, -29.0336)
  line L145 (-73.6515, -29.0336) -> (-72.6228, -31.3739)
  line L146 (-72.6228, -31.3739) -> (-66.4723, -28.6706)
  line L147 (-66.4723, -28.6706) -> (-66.0648, -29.5977)
  line L148 (-73.1395, -24.3893) -> (-73.1228, -24.4357)
  spline S132 degree 2 poles (-73.1228, -24.4357) (-73.1142, -24.5508) (-73.0442, -24.7815) (-72.9877, -24.9384) knots 0 0 0 1 2 2 2
  spline S133 degree 2 poles (-72.9877, -24.9384) (-72.8558, -25.3044) (-72.2768, -25.9097) (-71.8459, -26.122) knots 0 0 0 1 2 2 2
  line L149 (-71.8459, -26.122) -> (-68.029, -24.7472)
  line L150 (-68.029, -24.7472) -> (-67.7025, -25.6535)
  line L151 (-67.7025, -25.6535) -> (-73.0823, -27.5913)
  line L152 (-73.0823, -27.5913) -> (-73.4087, -26.685)
  line L153 (-73.4087, -26.685) -> (-72.607, -26.3962)
  spline S134 degree 2 poles (-72.607, -26.3962) (-73.2264, -26.0614) (-73.8524, -25.4533) (-73.9779, -25.1047) knots 0 0 0 1 2 2 2
  spline S135 degree 2 poles (-73.9779, -25.1047) (-74.0281, -24.9653) (-74.0667, -24.8217) (-74.0807, -24.7283) knots 0 0 0 1 2 2 2
  line L154 (-74.0807, -24.7283) -> (-73.1395, -24.3893)
  line L155 (-69.2341, -21.1468) -> (-68.9466, -22.0662)
  line L156 (-68.9466, -22.0662) -> (-74.404, -23.7729)
  line L157 (-74.404, -23.7729) -> (-74.6915, -22.8535)
  line L158 (-74.6915, -22.8535) -> (-69.2341, -21.1468)
  line L159 (-75.6194, -23.0725) -> (-75.2932, -24.1156)
  line L160 (-75.2932, -24.1156) -> (-76.2479, -24.4142)
  line L161 (-76.2479, -24.4142) -> (-76.5742, -23.371)
  line L162 (-76.5742, -23.371) -> (-75.6194, -23.0725)
  spline S136 degree 2 poles (-73.7561, -15.8886) (-72.3668, -15.5389) (-70.3929, -16.4494) (-70.1382, -17.4614) knots 0 0 0 1 2 2 2
  spline S137 degree 2 poles (-70.1382, -17.4614) (-70.0342, -17.8746) (-70.0661, -18.5576) (-70.1808, -18.9367) knots 0 0 0 1 2 2 2
  line L163 (-70.1808, -18.9367) -> (-67.8573, -18.3519)
  line L164 (-67.8573, -18.3519) -> (-67.6222, -19.2861)
  line L165 (-67.6222, -19.2861) -> (-75.2094, -21.1956)
  line L166 (-75.2094, -21.1956) -> (-75.4445, -20.2614)
  line L167 (-75.4445, -20.2614) -> (-74.8636, -20.1152)
  spline S138 degree 2 poles (-74.8636, -20.1152) (-75.2684, -19.8478) (-75.9016, -19.103) (-76.0267, -18.6059) knots 0 0 0 1 2 2 2
  spline S139 degree 2 poles (-76.0267, -18.6059) (-76.2664, -17.6538) (-75.0256, -16.2081) (-73.7561, -15.8886) knots 0 0 0 1 2 2 2
  spline S140 degree 2 poles (-73.4056, -16.8256) (-74.3578, -17.0652) (-75.2535, -17.9338) (-75.0832, -18.6104) knots 0 0 0 1 2 2 2
  spline S141 degree 2 poles (-75.0832, -18.6104) (-74.9837, -19.0057) (-74.4435, -19.6593) (-74.0852, -19.9193) knots 0 0 0 1 2 2 2
  line L168 (-74.0852, -19.9193) -> (-70.9353, -19.1266)
  spline S142 degree 2 poles (-70.9353, -19.1266) (-70.8536, -18.7176) (-70.853, -18.1634) (-70.9374, -17.8281) knots 0 0 0 1 2 2 2
  spline S143 degree 2 poles (-70.9374, -17.8281) (-71.1197, -17.1035) (-72.3876, -16.5693) (-73.4056, -16.8256) knots 0 0 0 1 2 2 2
  spline S144 degree 2 poles (-74.6235, -10.0137) (-73.1987, -9.7731) (-71.4147, -10.8809) (-71.2213, -12.0256) knots 0 0 0 1 2 2 2
  spline S145 degree 2 poles (-71.2213, -12.0256) (-71.0229, -13.2007) (-72.397, -14.8168) (-73.773, -15.0492) knots 0 0 0 1 2 2 2
  spline S146 degree 2 poles (-73.773, -15.0492) (-75.1856, -15.2878) (-76.9849, -14.1638) (-77.1762, -13.0313) knots 0 0 0 1 2 2 2
  spline S147 degree 2 poles (-77.1762, -13.0313) (-77.3695, -11.8866) (-76.0422, -10.2533) (-74.6235, -10.0137) knots 0 0 0 1 2 2 2
  spline S148 degree 2 poles (-74.4579, -10.994) (-75.5539, -11.1791) (-76.4847, -12.1567) (-76.3603, -12.8935) knots 0 0 0 1 2 2 2
  spline S149 degree 2 poles (-76.3603, -12.8935) (-76.2359, -13.6302) (-75.0346, -14.254) (-73.9386, -14.0689) knots 0 0 0 1 2 2 2
  spline S150 degree 2 poles (-73.9386, -14.0689) (-72.8731, -13.8889) (-71.9128, -12.9001) (-72.0372, -12.1634) knots 0 0 0 1 2 2 2
  spline S151 degree 2 poles (-72.0372, -12.1634) (-72.1606, -11.4327) (-73.3741, -10.811) (-74.4579, -10.994) knots 0 0 0 1 2 2 2
  line L169 (-72.3028, -4.177) -> (-72.2181, -5.1366)
  line L170 (-72.2181, -5.1366) -> (-72.7963, -5.1877)
  spline S152 degree 2 poles (-72.7963, -5.1877) (-72.5922, -5.3928) (-72.3174, -5.6971) (-72.1933, -5.9093) knots 0 0 0 1 2 2 2
  spline S153 degree 2 poles (-72.1933, -5.9093) (-72.0769, -6.1036) (-71.9338, -6.5311) (-71.9083, -6.8202) knots 0 0 0 1 2 2 2
  spline S154 degree 2 poles (-71.9083, -6.8202) (-71.867, -7.2877) (-72.185, -8.1092) (-72.5358, -8.4192) knots 0 0 0 1 2 2 2
  spline S155 degree 2 poles (-72.5358, -8.4192) (-72.8865, -8.7291) (-73.9666, -9.1344) (-74.6863, -9.198) knots 0 0 0 1 2 2 2
  spline S156 degree 2 poles (-74.6863, -9.198) (-75.4367, -9.2642) (-76.5658, -8.9734) (-77.0078, -8.6714) knots 0 0 0 1 2 2 2
  spline S157 degree 2 poles (-77.0078, -8.6714) (-77.4046, -8.3903) (-77.9067, -7.5482) (-77.9496, -7.0623) knots 0 0 0 1 2 2 2
  spline S158 degree 2 poles (-77.9496, -7.0623) (-77.9871, -6.6378) (-77.8523, -5.9874) (-77.6864, -5.6194) knots 0 0 0 1 2 2 2
  line L171 (-77.6864, -5.6194) -> (-80.1469, -5.8367)
  line L172 (-80.1469, -5.8367) -> (-80.2316, -4.8771)
  line L173 (-80.2316, -4.8771) -> (-72.3028, -4.177)
  line L174 (-73.6021, -5.2588) -> (-76.8929, -5.5494)
  spline S159 degree 2 poles (-76.8929, -5.5494) (-77.0337, -5.9213) (-77.1129, -6.4987) (-77.0841, -6.8247) knots 0 0 0 1 2 2 2
  spline S160 degree 2 poles (-77.0841, -6.8247) (-77.0189, -7.5628) (-75.8379, -8.3016) (-74.7922, -8.2093) knots 0 0 0 1 2 2 2
  spline S161 degree 2 poles (-74.7922, -8.2093) (-73.7834, -8.1202) (-72.7757, -7.3865) (-72.8382, -6.6791) knots 0 0 0 1 2 2 2
  spline S162 degree 2 poles (-72.8382, -6.6791) (-72.8713, -6.3039) (-73.2831, -5.5716) (-73.6021, -5.2588) knots 0 0 0 1 2 2 2
  line L175 (-72.3811, -1.2886) -> (-72.3491, -2.5109)
  line L176 (-72.3491, -2.5109) -> (-73.8059, -2.549)
  line L177 (-73.8059, -2.549) -> (-73.8379, -1.3267)
  line L178 (-73.8379, -1.3267) -> (-72.3811, -1.2886)
  line L179 (-72.3786, 1.3724) -> (-72.3904, 0.4092)
  line L180 (-72.3904, 0.4092) -> (-78.1081, 0.4795)
  line L181 (-78.1081, 0.4795) -> (-78.0962, 1.4427)
  line L182 (-78.0962, 1.4427) -> (-72.3786, 1.3724)
  line L183 (-79.0463, 1.5224) -> (-79.0597, 0.4295)
  line L184 (-79.0597, 0.4295) -> (-80.06, 0.4418)
  line L185 (-80.06, 0.4418) -> (-80.0466, 1.5347)
  line L186 (-80.0466, 1.5347) -> (-79.0463, 1.5224)
  spline S163 degree 2 poles (-75.0464, 7.7739) (-73.6172, 7.6754) (-72.0231, 6.1975) (-72.0949, 5.1564) knots 0 0 0 1 2 2 2
  spline S164 degree 2 poles (-72.0949, 5.1564) (-72.1242, 4.7314) (-72.3664, 4.0919) (-72.593, 3.7671) knots 0 0 0 1 2 2 2
  line L187 (-72.593, 3.7671) -> (-70.2028, 3.6023)
  line L188 (-70.2028, 3.6023) -> (-70.2691, 2.6413)
  line L189 (-70.2691, 2.6413) -> (-78.0743, 3.1795)
  line L190 (-78.0743, 3.1795) -> (-78.008, 4.1405)
  line L191 (-78.008, 4.1405) -> (-77.4105, 4.0993)
  spline S165 degree 2 poles (-77.4105, 4.0993) (-77.7124, 4.4791) (-78.0833, 5.3836) (-78.048, 5.8949) knots 0 0 0 1 2 2 2
  spline S166 degree 2 poles (-78.048, 5.8949) (-77.9805, 6.8744) (-76.3525, 7.8639) (-75.0464, 7.7739) knots 0 0 0 1 2 2 2
  spline S167 degree 2 poles (-75.0039, 6.7744) (-75.9834, 6.842) (-77.1044, 6.2941) (-77.1524, 5.598) knots 0 0 0 1 2 2 2
  spline S168 degree 2 poles (-77.1524, 5.598) (-77.1804, 5.1914) (-76.8696, 4.4024) (-76.6096, 4.0441) knots 0 0 0 1 2 2 2
  line L192 (-76.6096, 4.0441) -> (-73.3693, 3.8207)
  spline S169 degree 2 poles (-73.3693, 3.8207) (-73.1647, 4.1841) (-72.9922, 4.7107) (-72.9684, 5.0557) knots 0 0 0 1 2 2 2
  spline S170 degree 2 poles (-72.9684, 5.0557) (-72.917, 5.8011) (-73.9567, 6.7022) (-75.0039, 6.7744) knots 0 0 0 1 2 2 2
  spline S171 degree 2 poles (-71.5508, 10.2551) (-71.6548, 9.4778) (-72.6594, 8.7214) (-73.6204, 8.85) knots 0 0 0 1 2 2 2
  line L193 (-73.6204, 8.85) -> (-76.7602, 9.2702)
  line L194 (-76.7602, 9.2702) -> (-76.8462, 8.6275)
  line L195 (-76.8462, 8.6275) -> (-77.6357, 8.7332)
  line L196 (-77.6357, 8.7332) -> (-77.5497, 9.3758)
  line L197 (-77.5497, 9.3758) -> (-79.1777, 9.5937)
  line L198 (-79.1777, 9.5937) -> (-79.05, 10.5485)
  line L199 (-79.05, 10.5485) -> (-77.4219, 10.3306)
  line L200 (-77.4219, 10.3306) -> (-77.1868, 12.0872)
  line L201 (-77.1868, 12.0872) -> (-76.3973, 11.9815)
  line L202 (-76.3973, 11.9815) -> (-76.6324, 10.225)
  line L203 (-76.6324, 10.225) -> (-73.9332, 9.8637)
  spline S172 degree 2 poles (-73.9332, 9.8637) (-73.5048, 9.8064) (-73.0294, 9.7739) (-72.8135, 9.8509) knots 0 0 0 1 2 2 2
  spline S173 degree 2 poles (-72.8135, 9.8509) (-72.6246, 9.9129) (-72.3955, 10.2747) (-72.3512, 10.6052) knots 0 0 0 1 2 2 2
  spline S174 degree 2 poles (-72.3512, 10.6052) (-72.3201, 10.8378) (-72.4027, 11.2912) (-72.4325, 11.3948) knots 0 0 0 1 2 2 2
  line L204 (-72.4325, 11.3948) -> (-72.4251, 11.4499)
  line L205 (-72.4251, 11.4499) -> (-71.5682, 11.3352)
  spline S175 degree 2 poles (-71.5682, 11.3352) (-71.5308, 11.0561) (-71.5189, 10.4938) (-71.5508, 10.2551) knots 0 0 0 1 2 2 2
  line L206 (-69.7993, 19.2983) -> (-70.6899, 15.6892)
  line L207 (-70.6899, 15.6892) -> (-71.4453, 15.8756)
  line L208 (-71.4453, 15.8756) -> (-71.1139, 17.2185)
  line L209 (-71.1139, 17.2185) -> (-76.0719, 18.4421)
  line L210 (-76.0719, 18.4421) -> (-76.4033, 17.0991)
  line L211 (-76.4033, 17.0991) -> (-77.0808, 17.2663)
  spline S176 degree 2 poles (-77.0808, 17.2663) (-76.8929, 18.0277) (-77.147, 18.8537) (-77.7347, 19.0496) knots 0 0 0 1 2 2 2
  line L212 (-77.7347, 19.0496) -> (-77.5453, 19.817)
  line L213 (-77.5453, 19.817) -> (-70.8787, 18.1718)
  line L214 (-70.8787, 18.1718) -> (-70.5547, 19.4847)
  line L215 (-70.5547, 19.4847) -> (-69.7993, 19.2983)
  spline S177 degree 2 poles (-74.3688, 22.0702) (-74.9254, 22.2553) (-75.7305, 22.9263) (-75.9594, 23.3538) knots 0 0 0 1 2 2 2
  spline S178 degree 2 poles (-75.9594, 23.3538) (-76.1823, 23.7597) (-76.2496, 24.7516) (-76.1016, 25.197) knots 0 0 0 1 2 2 2
  spline S179 degree 2 poles (-76.1016, 25.197) (-75.936, 25.6951) (-75.3332, 26.3927) (-74.9175, 26.5864) knots 0 0 0 1 2 2 2
  spline S180 degree 2 poles (-74.9175, 26.5864) (-74.3943, 26.829) (-72.9688, 26.8107) (-71.9785, 26.4815) knots 0 0 0 1 2 2 2
  spline S181 degree 2 poles (-71.9785, 26.4815) (-71.082, 26.1835) (-69.6108, 25.2455) (-69.208, 24.6757) knots 0 0 0 1 2 2 2
  spline S182 degree 2 poles (-69.208, 24.6757) (-68.7838, 24.0727) (-68.5814, 22.704) (-68.8658, 21.8484) knots 0 0 0 1 2 2 2
  spline S183 degree 2 poles (-68.8658, 21.8484) (-68.9301, 21.6551) (-69.1172, 21.2292) (-69.2381, 21.0612) knots 0 0 0 1 2 2 2
  line L216 (-69.2381, 21.0612) -> (-70.1698, 21.3709)
  line L217 (-70.1698, 21.3709) -> (-70.1542, 21.4177)
  spline S184 degree 2 poles (-70.1542, 21.4177) (-70.043, 21.5174) (-69.7486, 21.9922) (-69.6609, 22.2559) knots 0 0 0 1 2 2 2
  spline S185 degree 2 poles (-69.6609, 22.2559) (-69.3454, 23.2052) (-70.2391, 24.706) (-71.374, 25.1679) knots 0 0 0 1 2 2 2
  spline S186 degree 2 poles (-71.374, 25.1679) (-71.2389, 24.6935) (-71.2323, 23.9104) (-71.3706, 23.4944) knots 0 0 0 1 2 2 2
  spline S187 degree 2 poles (-71.3706, 23.4944) (-71.5031, 23.0959) (-71.8989, 22.4922) (-72.2619, 22.2419) knots 0 0 0 1 2 2 2
  spline S188 degree 2 poles (-72.2619, 22.2419) (-72.6893, 21.9545) (-73.73, 21.8579) (-74.3688, 22.0702) knots 0 0 0 1 2 2 2
  spline S189 degree 2 poles (-72.5206, 25.575) (-73.2531, 25.8185) (-74.2685, 25.8566) (-74.6003, 25.7001) knots 0 0 0 1 2 2 2
  spline S190 degree 2 poles (-74.6003, 25.7001) (-74.9049, 25.5671) (-75.2267, 25.186) (-75.3124, 24.9282) knots 0 0 0 1 2 2 2
  spline S191 degree 2 poles (-75.3124, 24.9282) (-75.5111, 24.3305) (-74.8912, 23.3371) (-74.0826, 23.0683) knots 0 0 0 1 2 2 2
  spline S192 degree 2 poles (-74.0826, 23.0683) (-73.6255, 22.9164) (-72.9558, 22.9541) (-72.6591, 23.1418) knots 0 0 0 1 2 2 2
  spline S193 degree 2 poles (-72.6591, 23.1418) (-72.4444, 23.2787) (-72.1909, 23.7085) (-72.1013, 23.978) knots 0 0 0 1 2 2 2
  spline S194 degree 2 poles (-72.1013, 23.978) (-71.9981, 24.2886) (-71.9773, 25.0756) (-72.0694, 25.4055) knots 0 0 0 1 2 2 2
  spline S195 degree 2 poles (-72.0694, 25.4055) (-72.1377, 25.4347) (-72.3741, 25.5263) (-72.5206, 25.575) knots 0 0 0 1 2 2 2
  line L218 (-71.6805, 32.9875) -> (-66.9974, 27.4286)
  line L219 (-66.9974, 27.4286) -> (-67.4204, 26.4275)
  line L220 (-67.4204, 26.4275) -> (-72.2589, 32.2532)
  line L221 (-72.2589, 32.2532) -> (-73.7901, 28.63)
  line L222 (-73.7901, 28.63) -> (-74.6149, 28.9785)
  line L223 (-74.6149, 28.9785) -> (-72.7327, 33.4322)
  line L224 (-72.7327, 33.4322) -> (-71.6805, 32.9875)
  line L225 (-60.4517, 39.9205) -> (-63.2816, 41.637)
  spline S196 degree 2 poles (-63.2816, 41.637) (-63.6195, 41.842) (-64.227, 42.1382) (-64.4367, 42.1498) knots 0 0 0 1 2 2 2
  spline S197 degree 2 poles (-64.4367, 42.1498) (-64.6621, 42.171) (-65.0264, 41.9514) (-65.1962, 41.6716) knots 0 0 0 1 2 2 2
  spline S198 degree 2 poles (-65.1962, 41.6716) (-65.3499, 41.4182) (-65.3906, 40.6485) (-65.2807, 40.1629) knots 0 0 0 1 2 2 2
  spline S199 degree 2 poles (-65.2807, 40.1629) (-65.2036, 40.1234) (-64.9913, 40.009) (-64.854, 39.9258) knots 0 0 0 1 2 2 2
  line L226 (-64.854, 39.9258) -> (-61.6334, 37.9723)
  line L227 (-61.6334, 37.9723) -> (-62.1329, 37.1486)
  line L228 (-62.1329, 37.1486) -> (-64.9629, 38.8651)
  spline S200 degree 2 poles (-64.9629, 38.8651) (-65.3008, 39.0701) (-65.9083, 39.3664) (-66.1179, 39.378) knots 0 0 0 1 2 2 2
  spline S201 degree 2 poles (-66.1179, 39.378) (-66.3434, 39.3992) (-66.7077, 39.1796) (-66.8774, 38.8997) knots 0 0 0 1 2 2 2
  spline S202 degree 2 poles (-66.8774, 38.8997) (-67.0375, 38.6358) (-67.0604, 37.848) (-66.9682, 37.4165) knots 0 0 0 1 2 2 2
  line L229 (-66.9682, 37.4165) -> (-63.3146, 35.2004)
  line L230 (-63.3146, 35.2004) -> (-63.8142, 34.3768)
  line L231 (-63.8142, 34.3768) -> (-68.7032, 37.3422)
  line L232 (-68.7032, 37.3422) -> (-68.2037, 38.1659)
  line L233 (-68.2037, 38.1659) -> (-67.6651, 37.8392)
  spline S203 degree 2 poles (-67.6651, 37.8392) (-67.7919, 38.3566) (-67.7613, 39.2048) (-67.5307, 39.5849) knots 0 0 0 1 2 2 2
  spline S204 degree 2 poles (-67.5307, 39.5849) (-67.2681, 40.0178) (-66.4654, 40.4482) (-65.911, 40.3502) knots 0 0 0 1 2 2 2
  spline S205 degree 2 poles (-65.911, 40.3502) (-66.1007, 40.9781) (-66.0992, 41.9449) (-65.8495, 42.3568) knots 0 0 0 1 2 2 2
  spline S206 degree 2 poles (-65.8495, 42.3568) (-65.6573, 42.6735) (-65.1481, 43.0725) (-64.8111, 43.128) knots 0 0 0 1 2 2 2
  spline S207 degree 2 poles (-64.8111, 43.128) (-64.4709, 43.1889) (-63.6743, 43.0019) (-63.1727, 42.6976) knots 0 0 0 1 2 2 2
  line L234 (-63.1727, 42.6976) -> (-59.9521, 40.7441)
  line L235 (-59.9521, 40.7441) -> (-60.4517, 39.9205)
  line L236 (-55.172, 46.9479) -> (-57.7732, 48.9945)
  spline S208 degree 2 poles (-57.7732, 48.9945) (-58.0838, 49.2388) (-58.651, 49.6065) (-58.8577, 49.6434) knots 0 0 0 1 2 2 2
  spline S209 degree 2 poles (-58.8577, 49.6434) (-59.0789, 49.6918) (-59.4671, 49.5179) (-59.6695, 49.2607) knots 0 0 0 1 2 2 2
  spline S210 degree 2 poles (-59.6695, 49.2607) (-59.8528, 49.0277) (-59.9864, 48.2686) (-59.9361, 47.7733) knots 0 0 0 1 2 2 2
  spline S211 degree 2 poles (-59.9361, 47.7733) (-59.8644, 47.7247) (-59.6675, 47.5855) (-59.5413, 47.4862) knots 0 0 0 1 2 2 2
  line L237 (-59.5413, 47.4862) -> (-56.5809, 45.1571)
  line L238 (-56.5809, 45.1571) -> (-57.1766, 44.4)
  line L239 (-57.1766, 44.4) -> (-59.7778, 46.4466)
  spline S212 degree 2 poles (-59.7778, 46.4466) (-60.0884, 46.691) (-60.6556, 47.0587) (-60.8622, 47.0956) knots 0 0 0 1 2 2 2
  spline S213 degree 2 poles (-60.8622, 47.0956) (-61.0835, 47.1439) (-61.4717, 46.9701) (-61.6741, 46.7128) knots 0 0 0 1 2 2 2
  spline S214 degree 2 poles (-61.6741, 46.7128) (-61.865, 46.4702) (-61.9831, 45.691) (-61.9438, 45.2515) knots 0 0 0 1 2 2 2
  line L240 (-61.9438, 45.2515) -> (-58.5855, 42.6093)
  line L241 (-58.5855, 42.6093) -> (-59.1812, 41.8522)
  line L242 (-59.1812, 41.8522) -> (-63.6751, 45.3879)
  line L243 (-63.6751, 45.3879) -> (-63.0794, 46.145)
  line L244 (-63.0794, 46.145) -> (-62.5844, 45.7555)
  spline S215 degree 2 poles (-62.5844, 45.7555) (-62.6475, 46.2845) (-62.5145, 47.1227) (-62.2396, 47.4721) knots 0 0 0 1 2 2 2
  spline S216 degree 2 poles (-62.2396, 47.4721) (-61.9265, 47.87) (-61.0776, 48.2) (-60.5391, 48.0356) knots 0 0 0 1 2 2 2
  spline S217 degree 2 poles (-60.5391, 48.0356) (-60.6514, 48.6818) (-60.5328, 49.6414) (-60.235, 50.0199) knots 0 0 0 1 2 2 2
  spline S218 degree 2 poles (-60.235, 50.0199) (-60.0059, 50.3111) (-59.4521, 50.6454) (-59.1109, 50.6598) knots 0 0 0 1 2 2 2
  spline S219 degree 2 poles (-59.1109, 50.6598) (-58.7658, 50.679) (-57.9977, 50.3968) (-57.5367, 50.0341) knots 0 0 0 1 2 2 2
  line L245 (-57.5367, 50.0341) -> (-54.5763, 47.7049)
  line L246 (-54.5763, 47.7049) -> (-55.172, 46.9479)
  line L247 (-48.1845, 54.0684) -> (-48.8839, 53.406)
  line L248 (-48.8839, 53.406) -> (-49.2831, 53.8274)
  spline S220 degree 2 poles (-49.2831, 53.8274) (-49.3171, 53.5401) (-49.3848, 53.1357) (-49.474, 52.9066) knots 0 0 0 1 2 2 2
  spline S221 degree 2 poles (-49.474, 52.9066) (-49.554, 52.6947) (-49.8002, 52.317) (-50.0109, 52.1174) knots 0 0 0 1 2 2 2
  spline S222 degree 2 poles (-50.0109, 52.1174) (-50.3516, 51.7947) (-51.193, 51.5336) (-51.6537, 51.616) knots 0 0 0 1 2 2 2
  spline S223 degree 2 poles (-51.6537, 51.616) (-52.1145, 51.6984) (-53.103, 52.293) (-53.5999, 52.8176) knots 0 0 0 1 2 2 2
  spline S224 degree 2 poles (-53.5999, 52.8176) (-54.1179, 53.3645) (-54.5913, 54.4301) (-54.6293, 54.964) knots 0 0 0 1 2 2 2
  spline S225 degree 2 poles (-54.6293, 54.964) (-54.6554, 55.4496) (-54.3073, 56.3661) (-53.9531, 56.7016) knots 0 0 0 1 2 2 2
  spline S226 degree 2 poles (-53.9531, 56.7016) (-53.6438, 56.9946) (-53.0504, 57.293) (-52.659, 57.3916) knots 0 0 0 1 2 2 2
  line L249 (-52.659, 57.3916) -> (-54.3575, 59.1849)
  line L250 (-54.3575, 59.1849) -> (-53.6581, 59.8473)
  line L251 (-53.6581, 59.8473) -> (-48.1845, 54.0684)
  line L252 (-49.8393, 54.4147) -> (-52.1112, 56.8132)
  spline S227 degree 2 poles (-52.1112, 56.8132) (-52.4901, 56.6925) (-52.9917, 56.396) (-53.2293, 56.1709) knots 0 0 0 1 2 2 2
  spline S228 degree 2 poles (-53.2293, 56.1709) (-53.7673, 55.6613) (-53.6127, 54.2768) (-52.8908, 53.5147) knots 0 0 0 1 2 2 2
  spline S229 degree 2 poles (-52.8908, 53.5147) (-52.1944, 52.7795) (-50.9935, 52.4455) (-50.4779, 52.9338) knots 0 0 0 1 2 2 2
  spline S230 degree 2 poles (-50.4779, 52.9338) (-50.2045, 53.1929) (-49.8863, 53.9705) (-49.8393, 54.4147) knots 0 0 0 1 2 2 2
  line L253 (-46.3636, 55.5964) -> (-47.0993, 54.9746)
  line L254 (-47.0993, 54.9746) -> (-50.7906, 59.3416)
  line L255 (-50.7906, 59.3416) -> (-50.0549, 59.9634)
  line L256 (-50.0549, 59.9634) -> (-46.3636, 55.5964)
  line L257 (-50.6169, 60.7335) -> (-51.4516, 60.028)
  line L258 (-51.4516, 60.028) -> (-52.0974, 60.7919)
  line L259 (-52.0974, 60.7919) -> (-51.2627, 61.4975)
  line L260 (-51.2627, 61.4975) -> (-50.6169, 60.7335)
  spline S231 degree 2 poles (-43.1096, 58.9164) (-43.1511, 58.7767) (-43.2802, 58.2921) (-43.3721, 58.1065) knots 0 0 0 1 2 2 2
  spline S232 degree 2 poles (-43.3721, 58.1065) (-43.4922, 57.8454) (-43.7859, 57.4454) (-44.1307, 57.1848) knots 0 0 0 1 2 2 2
  spline S233 degree 2 poles (-44.1307, 57.1848) (-44.4115, 56.9726) (-45.079, 56.8009) (-45.4163, 56.8478) knots 0 0 0 1 2 2 2
  spline S234 degree 2 poles (-45.4163, 56.8478) (-45.7401, 56.8972) (-46.3788, 57.2814) (-46.6096, 57.5868) knots 0 0 0 1 2 2 2
  spline S235 degree 2 poles (-46.6096, 57.5868) (-46.9671, 58.0598) (-47.0744, 59.0313) (-46.7861, 59.5511) knots 0 0 0 1 2 2 2
  spline S236 degree 2 poles (-46.7861, 59.5511) (-46.5359, 60.0189) (-45.5921, 60.9412) (-45.0122, 61.4337) knots 0 0 0 1 2 2 2
  line L261 (-45.0122, 61.4337) -> (-45.1239, 61.5815)
  spline S237 degree 2 poles (-45.1239, 61.5815) (-45.325, 61.8475) (-45.737, 62.0547) (-45.9556, 62.0366) knots 0 0 0 1 2 2 2
  spline S238 degree 2 poles (-45.9556, 62.0366) (-46.1741, 62.0185) (-46.6424, 61.7574) (-46.869, 61.5861) knots 0 0 0 1 2 2 2
  spline S239 degree 2 poles (-46.869, 61.5861) (-47.135, 61.385) (-47.7351, 60.6838) (-47.9793, 60.2593) knots 0 0 0 1 2 2 2
  line L262 (-47.9793, 60.2593) -> (-48.0237, 60.2258)
  line L263 (-48.0237, 60.2258) -> (-48.6157, 61.009)
  spline S240 degree 2 poles (-48.6157, 61.009) (-48.4485, 61.2283) (-47.7671, 61.9755) (-47.3779, 62.2696) knots 0 0 0 1 2 2 2
  spline S241 degree 2 poles (-47.3779, 62.2696) (-46.905, 62.6271) (-46.148, 62.9671) (-45.7466, 62.9685) knots 0 0 0 1 2 2 2
  spline S242 degree 2 poles (-45.7466, 62.9685) (-45.3539, 62.9712) (-44.657, 62.5613) (-44.3331, 62.1327) knots 0 0 0 1 2 2 2
  line L264 (-44.3331, 62.1327) -> (-41.9762, 59.0144)
  line L265 (-41.9762, 59.0144) -> (-42.7447, 58.4336)
  line L266 (-42.7447, 58.4336) -> (-43.1096, 58.9164)
  line L267 (-43.5936, 59.5568) -> (-44.5505, 60.8228)
  spline S243 degree 2 poles (-44.5505, 60.8228) (-44.8078, 60.5897) (-45.577, 59.8767) (-45.7785, 59.6005) knots 0 0 0 1 2 2 2
  spline S244 degree 2 poles (-45.7785, 59.6005) (-46.0132, 59.2761) (-46.1181, 58.5853) (-45.8575, 58.2405) knots 0 0 0 1 2 2 2
  spline S245 degree 2 poles (-45.8575, 58.2405) (-45.5596, 57.8464) (-44.8147, 57.7825) (-44.391, 58.1027) knots 0 0 0 1 2 2 2
  spline S246 degree 2 poles (-44.391, 58.1027) (-44.0314, 58.3745) (-43.6748, 59.1316) (-43.5936, 59.5568) knots 0 0 0 1 2 2 2
  line L268 (-35.3726, 63.2205) -> (-37.0984, 66.0447)
  spline S247 degree 2 poles (-37.0984, 66.0447) (-37.3045, 66.382) (-37.7082, 66.9241) (-37.8891, 67.0307) knots 0 0 0 1 2 2 2
  spline S248 degree 2 poles (-37.8891, 67.0307) (-38.0796, 67.153) (-38.5041, 67.1252) (-38.7833, 66.9546) knots 0 0 0 1 2 2 2
  spline S249 degree 2 poles (-38.7833, 66.9546) (-39.0363, 66.8) (-39.4259, 66.135) (-39.5512, 65.6531) knots 0 0 0 1 2 2 2
  spline S250 degree 2 poles (-39.5512, 65.6531) (-39.5008, 65.5826) (-39.3647, 65.3835) (-39.281, 65.2465) knots 0 0 0 1 2 2 2
  line L269 (-39.281, 65.2465) -> (-37.3169, 62.0324)
  line L270 (-37.3169, 62.0324) -> (-38.1389, 61.5301)
  line L271 (-38.1389, 61.5301) -> (-39.8647, 64.3543)
  spline S251 degree 2 poles (-39.8647, 64.3543) (-40.0708, 64.6915) (-40.4744, 65.2337) (-40.6553, 65.3402) knots 0 0 0 1 2 2 2
  spline S252 degree 2 poles (-40.6553, 65.3402) (-40.8459, 65.4626) (-41.2704, 65.4348) (-41.5496, 65.2642) knots 0 0 0 1 2 2 2
  spline S253 degree 2 poles (-41.5496, 65.2642) (-41.8131, 65.1032) (-42.1951, 64.4138) (-42.3113, 63.9882) knots 0 0 0 1 2 2 2
  line L272 (-42.3113, 63.9882) -> (-40.0832, 60.3419)
  line L273 (-40.0832, 60.3419) -> (-40.9052, 59.8396)
  line L274 (-40.9052, 59.8396) -> (-43.8868, 64.7189)
  line L275 (-43.8868, 64.7189) -> (-43.0648, 65.2212)
  line L276 (-43.0648, 65.2212) -> (-42.7363, 64.6837)
  spline S254 degree 2 poles (-42.7363, 64.6837) (-42.6113, 65.2015) (-42.1948, 65.9409) (-41.8154, 66.1728) knots 0 0 0 1 2 2 2
  spline S255 degree 2 poles (-41.8154, 66.1728) (-41.3833, 66.4368) (-40.4727, 66.4505) (-40.0251, 66.1089) knots 0 0 0 1 2 2 2